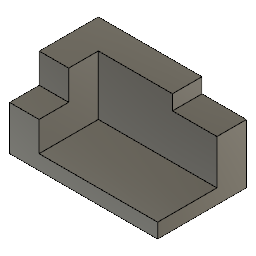
Tut1_P2 Exrude cut (Autodesk Fusion 360 design; units mm, degrees)
Autodesk Fusion 360 part; units mm, degrees
sketch "Sketch1" plane through (0, 0, 0) normal (0, 0, 1) x (1, 0, 0)
  line L0 (0, 0) -> (2540, 0)
  line L1 (2540, 0) -> (2540, 1524)
  line L2 (2540, 1524) -> (0, 1524)
  line L3 (0, 1524) -> (0, 0)
  line L4 (508, 0) -> (508, 1016)
  line L5 (508, 1016) -> (1778, 1016)
  line L6 (1778, 1016) -> (1778, 1524)
  line L7 (508, 508) -> (0, 508)
  line L8 (1778, 1016) -> (2540, 1016)
  dimension "d1" = 2540
  dimension "d2" = 1524
  dimension "d3" = 508
  dimension "d4" = 508
  dimension "d5" = 508
  dimension "d6" = 762
  measures "d1" distance of L0.start
  measures "d2" distance of L0.start
  measures "d3" distance of L3 L4
  measures "d4" distance of L0 L7
  measures "d5" distance of L2 L5
  measures "d6" distance of L1 L6
extrude "Extrude1" add sketch "Sketch1" along normal blind 254
sketch "Sketch2" plane through (0, 0, 254) normal (0, 0, 1) x (-1, 0, 0)
  line L0 (0, -1524) -> (0, 0)
  line L1 (0, 0) -> (-2540, 0)
  line L2 (-2540, 0) -> (-2540, -1524)
  line L3 (-2540, -1524) -> (0, -1524)
  line L4 (-508, 0) -> (-508, -1016)
  line L5 (-508, -1016) -> (-2540, -1016)
  dimension "d9" = 508
  dimension "d10" = 508
  measures "d9" distance of L0 L4
  measures "d10" distance of L3 L5
extrude "Extrude2" add sketch "Sketch2" along normal blind 508 contours L0 L1 L2 L3 L4 L5
sketch "Sketch3" plane through (0, 0, 762) normal (0, 0, 1) x (-1, 0, 0)
  line L0 (-508, -1016) -> (-2540, -1016)
  line L1 (-2540, -1016) -> (-2540, -1524)
  line L2 (-2540, -1524) -> (0, -1524)
  line L3 (0, -1524) -> (0, 0)
  line L4 (0, 0) -> (-508, 0)
  line L5 (-508, 0) -> (-508, -1016)
  line L6 (-508, -508) -> (0, -508)
  line L7 (-1778, -1016) -> (-1778, -1524)
  dimension "d13" = 762
  dimension "d14" = 508
  measures "d13" distance of L1 L7
  measures "d14" distance of L4 L6
extrude "Extrude3" add sketch "Sketch3" along normal blind 254 contours L0 L2 L3 L5 L6 L7 | L0 L1 L2 L7
sketch "Sketch4" plane through (0, 0, 1016) normal (0, 0, 1) x (-1, 0, 0)
  line L0 (-508, -1016) -> (-2540, -1016)
  line L1 (-2540, -1016) -> (-2540, -1524)
  line L2 (-2540, -1524) -> (0, -1524)
  line L3 (0, -1524) -> (0, -508)
  line L4 (0, -508) -> (-508, -508)
  line L5 (-508, -508) -> (-508, -1016)
  line L6 (-1778, -1524) -> (-1778, -1016)
  dimension "d17" = 762
  measures "d17" distance of L1 L6
extrude "Extrude4" add sketch "Sketch4" along normal blind 254 contours L0 L2 L3 L4 L5 L6
